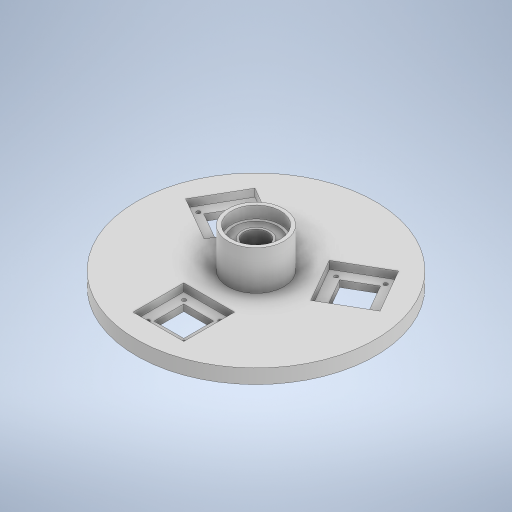
# Autodesk Inventor part: fixed_base
Saved by Autodesk Inventor 2024 (Build 280153000, 153)
## iProperties
Created: 2023-10-30
Part Number: fixed_base
Material: Generic
Document SubType Name: Modeling
Designer: MATEO
Density: 1 g/cm^3
Appearance: Default
Author: MATEO
Autodesk Inventor part; units mm, degrees
ref_plane "YZ Plane" through (0, 0, 0) normal (1, 0, 0) x (0, 1, 0)
ref_plane "XZ Plane" through (0, 0, 0) normal (0, 1, 0) x (-1, 0, 0)
ref_plane "XY Plane" through (0, 0, 0) normal (0, 0, 1) x (1, 0, 0)
sketch "Sketch1" plane through (0, 0, 0) normal (0, 1, 0) x (-1, 0, 0)
  circle A0 centre (0, 0) radius 100
  dimension "d0" = 200
  constraints: 1 centre point, 1 coincident
  measures "d0" diameter of A0
extrude "Extrusion1" add sketch "Sketch1" against normal blind 12
sketch "Sketch2" plane through (0, 0, 0) normal (0, 1, 0) x (1, 0, 0)
  circle A0 centre (0, 0) radius 23.5
  circle A1 centre (0, 0) radius 20.5
  dimension "d3" = 47
  dimension "d33" = 3
  constraints: 2 centre point, 1 coincident
  measures "d3" diameter of A0
  measures "d33" radial gap between concentric circles of A0 A1
extrude "Extrusion2" add sketch "Sketch2" along normal blind 33
sketch "Sketch7" plane through (0, 0, 0) normal (0, 1, 0) x (1, 0, 0)
  circle A0 centre (0, 0) radius 20.5 projected
  circle A1 centre (0, 0) radius 17.5
  circle A2 centre (0, 0) radius 10
  dimension "d37" = 35
  dimension "d40" = 20
  constraints: 2 centre point, 2 coincident
  measures "d37" diameter of A1
  measures "d40" diameter of A2
extrude "Extrusion7" add sketch "Sketch7" along normal blind 23 contours A0 | A1
sketch "Sketch8" plane through (0, 0, 0) normal (1, 0, 0) x (0, 1, 0)
  line L0 (0, -100) -> (0, 100) projected
  circle A0 centre (0, 5) radius 3.175
  line L1 (-4.445, 0) -> (4.445, 0) projected
  point P0 (0, 0)
  point P1 (0, 0)
  dimension "d41" = 6.35
  dimension "d42" = 5
  constraints: 1 centre point, 1 midpoint, 1 point on line
  measures "d41" diameter of A0
  measures "d42" distance of point (0, 0) A0.centre
revolve "Revolution1" cut sketch "Sketch8" angle 360 about axis through (0, -10, 0) along (0, 1, 0)
sketch "Sketch9" plane through (0, 0, 0) normal (1, 0, 0) x (0, 1, 0)
  circle A0 centre (23, 15) radius 3.175
  line L0 (23, 10) -> (23, -10) projected
  line L1 (23, 20.5) -> (23, -20.5) projected
  line L2 (-5.235, 0) -> (31.41, 0) projected
  point P0 (0, 0)
  point P1 (23, 0)
  point P2 (23, 11.825)
  point P3 (23, 18.175)
  dimension "d44" = 6.35
  dimension "d45" = 15
  constraints: 1 centre point, 1 midpoint, 1 point on line
  measures "d44" diameter of A0
  measures "d45" distance of point (23, 0) A0.centre
revolve "Revolution2" cut sketch "Sketch9" angle 360 about axis through (0, -10, 0) along (0, 1, 0) picked at (21.9494, 14.8724) contours L1 A0
sketch "Sketch10" plane through (0, 0, 0) normal (0, 1, 0) x (1, 0, 0)
  line L0 (-15.2, -45) -> (15.2, -45) construction
  line L1 (15.2, -45) -> (15.2, -75.4) construction
  line L2 (15.2, -75.4) -> (-15.2, -75.4) construction
  line L3 (-15.2, -75.4) -> (-15.2, -45) construction
  circle A0 centre (-15.2, -45) radius 1.6
  circle A1 centre (15.2, -45) radius 1.6
  circle A2 centre (-15.2, -75.4) radius 1.6
  circle A3 centre (15.2, -75.4) radius 1.6
  point P0 (0, 0)
  point P1 (0, -45)
  point P2 (15.2, -60.2)
  dimension "d47" = 30.4
  dimension "d48" = 30.4
  dimension "d49" = 3.2
  dimension "d52" = 30.4
  dimension "d55" = 30.4
  dimension "d58" = 45
  constraints: 8 end point, 4 centre point, 2 horizontal, 2 midpoint, 2 parallel, 1 coincident, 1 perpendicular, 1 vertical, 1 vertical alignment, 6 other
  measures "d47" distance of L1.end L2.end
  measures "d48" distance of L0.end L1.end
  measures "d49" diameter of A0
  measures "d52" distance of A0.centre A1.centre
  measures "d55" distance of A0.centre A2.centre
  measures "d58" distance of point (0, 0) point (0, -45)
extrude "Extrusion8" cut sketch "Sketch10" against normal through all
pattern_circular "Circular Pattern2" count 3 over 360 about axis through (0, 0, 0) along (0, -1, 0) of "Extrusion8"
sketch "Sketch11" plane through (0, 0, 0) normal (0, 1, 0) x (1, 0, 0)
  line L0 (-21.25, -39.2) -> (21.25, -39.2)
  line L1 (21.25, -39.2) -> (21.25, -81.7)
  line L2 (21.25, -81.7) -> (-21.25, -81.7)
  line L3 (-21.25, -81.7) -> (-21.25, -39.2)
  point P0 (0, 0)
  point P1 (0, -39.2)
  dimension "d64" = 42.5
  dimension "d65" = 42.5
  dimension "d66" = 39.2
  constraints: 8 end point, 2 parallel, 1 horizontal, 1 midpoint, 1 perpendicular, 1 vertical alignment
  measures "d64" distance of L1.end L2.end
  measures "d65" distance of L0.end L1.end
  measures "d66" distance from line of point (0, 0) L0
extrude "Extrusion9" cut sketch "Sketch11" against normal blind 6.5
pattern_circular "Circular Pattern3" count 3 over 360 about axis through (0, 0, 0) along (0, -1, 0) of "Extrusion9"
sketch "Sketch12" plane through (0, -6.5, 0) normal (0, 1, 0) x (1, 0, 0)
  line L0 (-12.5, -47.95) -> (12.5, -47.95)
  line L1 (12.5, -47.95) -> (12.5, -72.95)
  line L2 (12.5, -72.95) -> (-12.5, -72.95)
  line L3 (-12.5, -72.95) -> (-12.5, -47.95)
  line L4 (-21.25, -39.2) -> (21.25, -39.2) projected
  line L5 (21.25, -39.2) -> (21.25, -81.7) projected
  point P0 (0, 0)
  point P1 (0, -47.95)
  point P2 (0, -39.2)
  point P3 (12.5, -60.45)
  point P4 (21.25, -60.45)
  dimension "d72" = 25
  dimension "d73" = 25
  constraints: 8 end point, 4 midpoint, 2 parallel, 1 horizontal, 1 horizontal alignment, 1 perpendicular, 1 vertical alignment
  measures "d72" distance of L1.end L2.end
  measures "d73" distance of L0.end L1.end
extrude "Extrusion10" cut sketch "Sketch12" against normal through all
pattern_circular "Circular Pattern4" count 3 over 360 about axis through (0, 0, 0) along (0, -1, 0) of "Extrusion10"
body "Solid1"
